Autodesk Inventor part; units mm, degrees
(part 2 of 2)
sketch "스케치33" plane through (11.5034, 0, 0) normal (1, 0, 0) x (0, 1, 0)
  line L0 (0, 0) -> (58.4923, 0)
  line L1 (29.4, -4.4) -> (20.6, -4.4)
  line L2 (20.6, -4.4) -> (20.6, 4.4)
  line L3 (20.6, 4.4) -> (29.4, 4.4)
  line L4 (29.4, 4.4) -> (29.4, -4.4)
  circle A0 centre (25, 0) radius 3.5
  line L5 (25, -4.4) -> (25, 4.4) construction
  line L6 (29.4, 0) -> (20.6, 0) construction
  line L7 (0, 0) -> (25, 0)
  point P0 (29.394, 0.0017)
  dimension "d132" = 8.8
  dimension "d133" = 8.8
  dimension "d134" = 7
  dimension "d135" = 25
  constraints: 16 end point, 4 midpoint, 2 horizontal, 2 parallel, 1 centre point, 1 coincident, 1 perpendicular, 1 point on line
  measures "d132" distance of L2.end L3.end
  measures "d133" distance of L1.end L2.end
  measures "d134" diameter of A0
  measures "d135" distance of L0.start L7.end
extrude "돌출18" cut sketch "스케치33" along normal blind 10 contours L0 A0 | L0 A0
extrude "돌출19" cut sketch "스케치33" along normal blind 6.5
extrude "돌출20" add sketch "스케치33" along normal blind 3 contours A0 L0 L2 L3 L4 | L0 L4 L1 L2 A0
extrude "돌출21" cut sketch "스케치33" along normal blind 1 contours A0 L0 L2 L3 L4 | L0 L4 L1 L2 A0
ref_plane "작업 평면6" through (23.2534, 0, 0) normal (1, 0, 0) x (0, 1, 0)
sketch "스케치34" plane through (23.2534, 0, 0) normal (1, 0, 0) x (0, 1, 0)
  line L0 (-7.2232, 8.7062) -> (-7.2232, -8.7062) projected
  line L1 (-7.2232, 0) -> (51.7499, 0)
  line L2 (17, -25) -> (17, 25)
  line L3 (17.5, 2.5) -> (17.5, -2.5) projected
  circle A0 centre (25, 0) radius 3.5 construction
  circle A1 centre (17, 25) radius 5
  circle A2 centre (17, -25) radius 5
  point P0 (0, 0)
  point P1 (17.5, 0)
  dimension "d143" = 50
  dimension "d146" = 25
  dimension "d147" = 8
  dimension "d148" = 10
  dimension "d149" = 10
  constraints: 4 end point, 2 centre point, 2 coincident, 2 midpoint, 1 horizontal, 1 vertical
  measures "d143" distance of L2.start L2.end
  measures "d146" distance from line of L1 L2.end
  measures "d147" distance from line of L2 A0.centre
  measures "d148" diameter of A1
  measures "d149" diameter of A2
extrude "돌출22" add sketch "스케치34" along normal blind 9.5
sketch "스케치35" plane through (23.2534, 0, 0) normal (-1, 0, 0) x (0, 0, 1)
  arc A0 (24.5711, 12.0184) -> (24.5711, 21.9816) centre (25, 17) ccw projected
  arc A1 (-24.538, 21.9786) -> (-24.538, 12.0214) centre (-25, 17) ccw projected
  circle A2 centre (-25, 17) radius 2.6
  circle A3 centre (25, 17) radius 2.6
  point P0 (0, 0)
  dimension "d152" = 5.2
  dimension "d153" = 5.2
  constraints: 2 centre point, 2 coincident
  measures "d152" diameter of A2
  measures "d153" diameter of A3
extrude "돌출23" cut sketch "스케치35" against normal blind 9
sketch "스케치36" plane through (32.7534, 0, 0) normal (1, 0, 0) x (0, 0, -1)
  circle A0 centre (25, 17) radius 5 projected
  circle A1 centre (-25, 17) radius 5 projected
  circle A2 centre (-25, 17) radius 3
  circle A3 centre (25, 17) radius 3
  point P0 (0, 0)
  point P1 (29.5051, 14.8311)
  point P2 (29.5051, 19.1689)
  point P3 (-29.5564, 19.059)
  point P4 (-29.5564, 14.941)
  dimension "d156" = 6
  dimension "d157" = 6
  constraints: 2 centre point, 2 coincident
  measures "d156" diameter of A2
  measures "d157" diameter of A3
extrude "돌출24" cut sketch "스케치36" against normal blind 1 contours A2 | A3
sketch "스케치37" plane through (23.2534, 0, 0) normal (-1, 0, 0) x (0, 0, 1)
  arc A0 (-24.538, 19.5586) -> (-24.538, 14.4414) centre (-25, 17) ccw projected
  arc A1 (24.5711, 14.4356) -> (24.5711, 19.5644) centre (25, 17) ccw projected
  circle A2 centre (25, 17) radius 2.6 projected
  arc A3 (24.5711, 14.4356) -> (24.5711, 19.5644) centre (25, 17) ccw projected
  arc A4 (24.5711, 19.5644) -> (24.5711, 14.4356) centre (25, 17) ccw projected
  circle A5 centre (-25, 17) radius 2.6 projected
  arc A6 (-24.538, 14.4414) -> (-24.538, 19.5586) centre (-25, 17) ccw projected
  arc A7 (-24.538, 19.5586) -> (-24.538, 14.4414) centre (-25, 17) ccw projected
  point P0 (0, 0)
  point P1 (24.5711, 19.5644)
extrude "돌출25" cut sketch "스케치37" along normal blind 8
delete faces "면 삭제4" heal yes whole lump no faces at (24.3815, 16.837, 29.9973) (23.2534, 12.831, 25.1978)
delete faces "면 삭제5" heal yes whole lump no faces at (23.2534, 21.1465, -25.4721) (24.391, 16.8729, -29.9984)
sketch "스케치38" plane through (32.8721, 3.2182, 40) normal (-0.8485981, 0, 0.529038) x (0.529038, 0, 0.8485981)
  ellipse E0 centre (-17.6762, 13.7818) end of major axis (-20.7401, 13.7818) minor radius 2.6 projected
  ellipse E1 centre (-17.6762, 13.7818) end of major axis (-13.4955, 13.7818) minor radius 3.5321
  line L0 (-11.5892, 14.7818) -> (-24.8151, 14.7818) projected
  point P0 (-51.3345, -3.2182)
  constraints: 1 centre point, 1 coincident, 2 other
extrude "돌출26" cut sketch "스케치38" against normal blind 1
mirror "미러2" about plane through (0, 0, 0) normal (0, 0, 1) of "돌출26"
delete faces "면 삭제6" heal yes whole lump no faces at (12.17, 20.6, 0) (12.5034, 25.1406, -4.0915)
ref_plane "작업 평면7" through (11.5034, 25, 0) normal (0, -1, 0) x (1, 0, 0)
sketch "스케치39" plane through (11.5034, 25, 0) normal (0, -1, 0) x (1, 0, 0)
  line L0 (-3.8282, 0) -> (9.2324, 0)
  arc A0 (3.028, 10.5808) -> (3.0393, -10.5989) centre (20, 0) ccw projected
  arc A1 (1.6697, 5) -> (1.6697, -5) centre (20, 0) ccw
  line L1 (0.6351, 5) -> (1.6697, 5)
  line L2 (1.6697, -5) -> (0.6351, -5)
  line L3 (0.6351, 5) -> (-6.0591, 5)
  line L4 (-6.0591, 5) -> (-6.3381, 0)
  line L5 (-6.3381, 0) -> (-3.8282, 0)
  point P0 (-11.5034, 0)
  point P1 (0, 0)
  point P2 (1, 0)
  dimension "d164" = 1
  dimension "d165" = 10
  dimension "d166" = 5
  constraints: 12 end point, 6 horizontal, 4 point on circle, 1 centre point
  measures "d164" radial gap between concentric circles of A0 A1
  measures "d165" distance between parallel lines of L1 L2
  measures "d166" distance between parallel lines of L0 L1
revolve "회전6" cut sketch "스케치39" angle 360 about axis through (7.6752, 25, 0) along (1, 0, 0) contours L5 L4 L3 A0 L0 | A0 L1 A1 L0
sketch "스케치40" plane through (47.9273, 45, 40) normal (-0.3090861, 0.9510341, 0) x (0.9510341, 0.3090861, 0)
  line L0 (-15.8053, 79.9682) -> (0, 79.9702) projected
  line L1 (-14.5159, 74.9686) -> (-0.7921, 74.9703) construction
  line L2 (-0.7921, 5) -> (-14.5375, 5) projected
  line L3 (0, 0) -> (-15.8303, 0) projected
  line L4 (-15.8303, 0) -> (-35.1153, 29.4192) projected
  line L5 (-14.5375, 5) -> (-32.2788, 32.0644) projected
  line L6 (-35.1034, 50.5989) -> (-15.8053, 79.9682) projected
  line L7 (-32.2699, 47.9491) -> (-14.5159, 74.9686) projected
  ellipse E0 centre (-17.2695, 40) end of major axis (-38.2992, 40) minor radius 20 (-35.1034, 50.5989) -> (-35.1153, 29.4192) ccw projected
  ellipse E1 centre (-18.8945, 40) end of major axis (-3.1222, 40) minor radius 15 (-32.2699, 47.9491) -> (-32.2788, 32.0644) ccw projected
  line L8 (-0.7921, 74.9703) -> (-0.7921, 5) construction
  line L9 (-0.7921, 74.9703) -> (-0.7921, 5) construction
  line L10 (-12.3767, 9) -> (-4.7921, 9)
  line L11 (-4.7921, 9) -> (-4.7921, 70.9698)
  line L12 (-4.7921, 70.9698) -> (-12.3578, 70.9688)
  line L13 (-12.3578, 70.9688) -> (-28.927, 45.7526)
  line L14 (-28.9335, 34.2574) -> (-12.3767, 9)
  line L15 (-30.6062, 33.1609) -> (-13.4571, 7)
  line L16 (-13.4571, 7) -> (-2.7921, 7)
  line L17 (-2.7921, 7) -> (-2.7921, 72.97)
  line L18 (-2.7921, 72.97) -> (-13.4369, 72.9687)
  line L19 (-13.4369, 72.9687) -> (-30.5985, 46.8509)
  line L20 (-38.2992, 39.985) -> (5.1712, 39.985)
  line L21 (-2.7921, 7) -> (-33.3613, 38.5943)
  ellipse E2 centre (-20.4414, 40) end of major axis (-20.4414, 55) minor radius 14.2655 (-34.0794, 44.4) -> (-34.0794, 35.6) ccw projected
  line L22 (-2.7921, 72.97) -> (-33.3613, 41.3757)
  arc A0 (-33.3613, 41.3757) -> (-33.3613, 38.5943) centre (-31.924, 39.985) ccw
  spline S0 degree 5 poles (-28.927, 45.7526) (-29.5959, 44.7347) (-30.1226, 43.6233) (-30.4849, 42.4417) (-30.8473, 40.0059) (-30.4876, 37.5697) (-30.1267, 36.3878) (-29.6012, 35.2759) (-28.9335, 34.2573) knots 0 0 0 0 0 0 0.500015 0.500015 0.500015 1 1 1 1 1 1
  spline S1 degree 5 poles (-30.5985, 46.8509) (-31.3949, 45.6388) (-32.021, 44.3148) (-32.4509, 42.9074) (-32.881, 40.0071) (-32.4542, 37.1062) (-32.0259, 35.6984) (-31.4013, 34.3737) (-30.6062, 33.1609) knots 0 0 0 0 0 0 0.50001 0.50001 0.50001 1 1 1 1 1 1
  point P0 (-59.4893, 40)
  point P1 (-34.7069, 39.985)
  dimension "d170" = 2
  dimension "d168" = 4
  dimension "d176" = 2
  constraints: 28 end point, 3 parallel, 3 point on line, 2 point on circle, 2 tangent, 1 centre point, 1 horizontal, 1 vertical, 18 other
  measures "d168" distance between parallel lines of L2 L10
  measures "d176" radius of A0
extrude "돌출27" cut sketch "스케치40" against normal blind 2 contours L21 S1 L20 S0 L14 | L14 S0 L20 L11 L21 | L11 L20 L17 L21 | L21 A0 L20 S1 | L20 S0 L13 L22 L11 | L11 L22 L17 L20 | L20 S1 L22 L13 S0 | L20 A0 L22 S1
sketch "스케치42" plane through (48.5454, 43.0979, 40) normal (-0.3090861, 0.9510341, 0) x (0.9510341, 0.3090861, 0)
  line L0 (-2.7921, 7) -> (-33.3613, 38.5943) projected
  line L1 (-2.7921, 7) -> (-33.3613, 38.5943) projected
  line L2 (-2.7921, 72.97) -> (-2.7921, 7) projected
  line L3 (-33.3613, 41.3757) -> (-2.7921, 72.97) projected
  arc A0 (-33.3613, 41.3757) -> (-33.3613, 38.5943) centre (-31.924, 39.985) ccw projected
  line L4 (-4.2921, 10.7075) -> (-32.2833, 39.6373)
  arc A1 (-32.2833, 40.3327) -> (-32.2833, 39.6373) centre (-31.924, 39.985) ccw
  line L5 (-32.2833, 40.3327) -> (-4.2921, 69.2626)
  line L6 (-4.2921, 69.2626) -> (-4.2921, 10.7075)
  point P0 (-59.4893, 40)
  dimension "d177" = 1.5
  constraints: 6 end point, 2 point on circle, 1 centre point, 3 other
  measures "d177" distance between parallel lines of L2 L6
extrude "돌출29" cut sketch "스케치42" against normal blind 8 contours L4 A1 L5 L6
sketch "스케치43" plane through (78.1056, 18, 35) normal (0, 1, 0) x (1, 0, 0)
  line L0 (-12.6022, 29) -> (-37.6022, 29) projected
  line L1 (-37.6022, 29) -> (-37.6022, 24) projected
  line L2 (-37.6022, 24) -> (-12.6022, 24) projected
  line L3 (-12.6022, 24) -> (-12.6022, 29) projected
  line L4 (-37.6022, 41) -> (-12.6022, 41) projected
  line L5 (-12.6022, 41) -> (-12.6022, 46) projected
  line L6 (-12.6022, 46) -> (-37.6022, 46) projected
  line L7 (-37.6022, 46) -> (-37.6022, 41) projected
  line L8 (-37.6022, 24) -> (-12.6022, 24) projected
  line L9 (-12.6022, 46) -> (-37.6022, 46)
  line L10 (-37.6022, 46) -> (-37.6022, 24)
  line L11 (-37.6022, 24) -> (-12.6022, 24)
  line L12 (-12.6022, 24) -> (-12.6022, 46)
  line L13 (-35.1022, 26.5) -> (-35.1022, 43.5)
  line L14 (-35.1022, 43.5) -> (-15.1022, 43.5)
  line L15 (-15.1022, 43.5) -> (-15.1022, 26.5)
  line L16 (-15.1022, 26.5) -> (-35.1022, 26.5)
  point P0 (-78.1056, 35)
  dimension "d180" = 2.5
  constraints: 16 end point, 4 coincident, 4 parallel, 2 perpendicular, 1 horizontal, 3 other
  measures "d180" distance between parallel lines of L10 L13
hole "구멍2" at (43.0034, 18, 8.5) at (63.0034, 18, 8.5) at (63.0034, 18, -8.5) at (43.0034, 18, -8.5) direction (0, -1, 0) diameter 2.5 depth 8 tip angle 118
ref_plane "작업 평면8" through (77.9273, 8, 40) normal (0, -1, 0) x (1, 0, 0)
sketch "스케치45" plane through (77.9273, 8, 40) normal (0, -1, 0) x (1, 0, 0)
  line L0 (-42.2802, -5) -> (0.1783, -5) projected
  line L1 (-17.4239, -29) -> (-37.4239, -29)
  line L2 (-37.4239, -29) -> (-37.4239, -5)
  line L3 (-37.4239, -5) -> (-17.4239, -5)
  line L4 (-17.4239, -5) -> (-17.4239, -29)
  line L5 (-15.4243, 0) -> (-15.4243, -5) projected
  line L6 (-37.4239, -34) -> (-37.4239, -29) projected
  line L7 (-37.4239, -29) -> (-12.4239, -29) projected
  point P0 (-77.9273, -40)
  point P1 (-17.4239, -5)
  dimension "d196" = 20
  dimension "d198" = 0
  dimension "d199" = 0
  constraints: 8 end point, 2 parallel, 1 horizontal, 1 perpendicular, 1 point on line
  measures "d196" distance between parallel lines of L2 L4
  measures "d198" distance between parallel lines of L6 L2
  measures "d199" distance between parallel lines of L1 L7
extrude "돌출30" add sketch "스케치45" along normal up to next
sketch "스케치46" plane through (77.9273, 0, 40) normal (0, 0, 1) x (1, 0, 0)
  line L0 (-17.4239, 8) -> (-37.4239, 8) projected
  line L1 (-27.4239, 8) -> (-27.4239, 30.8064) construction
  line L2 (-35.9239, 9.6) -> (-18.9239, 9.6)
  line L3 (-18.9239, 9.6) -> (-18.9239, 8)
  line L4 (-18.9239, 8) -> (-35.9239, 8)
  line L5 (-35.9239, 8) -> (-35.9239, 9.6)
  line L6 (-31.9239, 12.2) -> (-22.9239, 12.2)
  line L7 (-22.9239, 12.2) -> (-22.9239, 9.6)
  line L8 (-22.9239, 9.6) -> (-31.9239, 9.6)
  line L9 (-31.9239, 9.6) -> (-31.9239, 12.2)
  line L10 (-27.4239, 8) -> (-27.4239, 12.295) construction
  line L11 (-27.4239, 9.6) -> (-27.4239, 12.2) construction
  point P0 (-77.9273, 0)
  point P1 (-27.4239, 9.6)
  point P2 (-31.9239, 9.6)
  dimension "d200" = 17
  dimension "d201" = 1.6
  dimension "d202" = 9
  dimension "d203" = 2.6
  constraints: 22 end point, 5 midpoint, 4 parallel, 2 coincident, 2 horizontal, 2 perpendicular, 2 vertical, 1 point on line
  measures "d200" distance of L3.end L4.end
  measures "d201" distance of L2.end L3.end
  measures "d202" distance of L7.end L8.end
  measures "d203" distance of L6.end L7.end
extrude "돌출31" cut sketch "스케치46" against normal blind 10
sketch "스케치48" plane through (77.9273, 0, 40) normal (0, -1, 0) x (1, 0, 0)
  line L0 (79.5042, -13.4713) -> (131.2352, -13.4713)
  line L1 (131.2352, -13.4713) -> (131.2352, -67.3578)
  line L2 (131.2352, -67.3578) -> (79.5042, -67.3578)
  line L3 (79.5042, -67.3578) -> (79.5042, -13.4713)
  arc A0 (109.7596, -29.4837) -> (109.6919, -50.5368) centre (106.5334, -40) ccw projected
  arc A1 (112.4054, -49.3016) -> (112.3603, -30.6701) centre (106.5334, -40) ccw projected
  circle A2 centre (106.5334, -40) radius 11 projected
  point P0 (-77.9273, -40)
  constraints: 8 end point, 2 parallel, 1 horizontal, 1 perpendicular
extrude "돌출33" cut sketch "스케치48" along normal blind 21 and the other way blind 5 contours A2 A1 A0 keep common part
delete faces "면 삭제8" heal yes whole lump no faces at (189.4206, 1.6667, 9.7254) (188.5237, 3.3333, -10.125)
sketch "스케치49" plane through (184.4606, 5, 0) normal (0, 1, 0) x (1, 0, 0)
  line L0 (0, 0) -> (0, 22.0992)
  point P0 (-184.4606, 0)
  constraints: 2 end point, 1 vertical
ref_plane "작업 평면9" through (184.4606, 5, 0) normal (0, 0, -1) x (-1, 0, 0)
equation "\"d82\" = 0.5 * d81"
